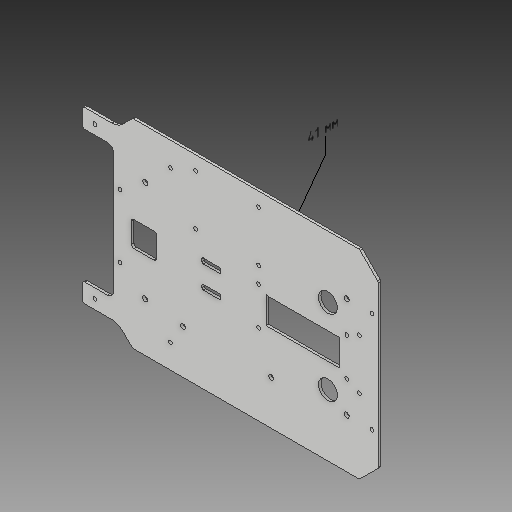
# Autodesk Inventor part: baseUp
Saved by Autodesk Inventor 2019 (Build 230136000, 136)
## iProperties
Created: 2018-05-21
Part Number: baseUp
Material: Типовые
Document SubType Name: Modeling
Designer: olege
Density: 1 g/cm^3
Appearance: По умолчанию
Mass: 63.0766 g
Surface Area: 659.094 cm^2
Volume: 63.0766 cm^3
Author: olege
Autodesk Inventor part; units mm, degrees
ref_plane "YZ Plane" through (0, 0, 0) normal (1, 0, 0) x (0, 1, 0)
ref_plane "XZ Plane" through (0, 0, 0) normal (0, 1, 0) x (-1, 0, 0)
sketch "Эскиз1" plane through (0, 0, 0) normal (0, 0, 1) x (1, 0, 0)
  line L0 (105, -79) -> (-105, -79)
  line L1 (-105, -79) -> (-105, 79)
  line L2 (-105, 79) -> (105, 79)
  line L3 (105, 79) -> (105, -79)
  line L4 (105, -79) -> (-105, 79) construction
  line L5 (-105, -79) -> (105, 79) construction
  point P0 (0, 0)
  dimension "d0" = 210
  dimension "d1" = 158
  constraints: 12 end point, 2 midpoint, 2 parallel, 1 horizontal, 1 perpendicular
  measures "d0" distance of L1.end L2.end
  measures "d1" distance of L0.end L1.end
extrude "Выдавливание1" add sketch "Эскиз1" along normal blind 2
chamfer "Фаска1" distance 15 angle 45 4 edges at (105, -79, 1) (-105, -79, 1) (-105, 79, 1) (105, 79, 1)
fillet "Сопряжение1" radius 2 8 edges at (90, 79, 1) (105, 64, 1) (105, -64, 1) (90, -79, 1) (-90, -79, 1) (-105, -64, 1) (-90, 79, 1) (-105, 64, 1)
sketch "Эскиз2" plane through (0, 0, 2) normal (0, 0, 1) x (1, 0, 0)
  line L0 (-100, 40) -> (100, 40) construction
  line L1 (100, 40) -> (100, -40) construction
  line L2 (100, -40) -> (-100, -40) construction
  line L3 (-100, -40) -> (-100, 40) construction
  line L4 (-100, 40) -> (100, -40) construction
  line L5 (100, 40) -> (-100, -40) construction
  circle A0 centre (100, -40) radius 1.5
  circle A1 centre (100, 40) radius 1.5
  point P0 (0, 0)
  dimension "d8" = 200
  dimension "d9" = 80
  dimension "d10" = 3
  dimension "d13" = 3
  constraints: 12 end point, 2 centre point, 2 coincident, 2 midpoint, 2 parallel, 1 horizontal, 1 perpendicular
  measures "d8" distance of L1.end L2.end
  measures "d9" distance of L0.end L1.end
  measures "d10" diameter of A0
  measures "d13" diameter of A1
extrude "фонарь" cut sketch "Эскиз2" against normal blind 2
sketch "Эскиз3" plane through (0, 0, 2) normal (0, 0, 1) x (1, 0, 0)
  line L0 (-90, 20) -> (90, 20) construction
  line L1 (90, 20) -> (90, -20) construction
  line L2 (90, -20) -> (-90, -20) construction
  line L3 (-90, -20) -> (-90, 20) construction
  line L4 (-90, 20) -> (90, -20) construction
  line L5 (90, 20) -> (-90, -20) construction
  circle A0 centre (90, -20) radius 1.5
  circle A1 centre (90, 20) radius 1.5
  point P0 (0, 0)
  dimension "d16" = 180
  dimension "d17" = 40
  dimension "d18" = 3
  dimension "d19" = 3
  constraints: 12 end point, 2 centre point, 2 coincident, 2 midpoint, 2 parallel, 1 horizontal, 1 perpendicular
  measures "d16" distance of L1.end L2.end
  measures "d17" distance of L0.end L1.end
  measures "d18" diameter of A0
  measures "d19" diameter of A1
extrude "камера" cut sketch "Эскиз3" against normal blind 2
sketch "Эскиз4" plane through (0, 0, 2) normal (0, 0, 1) x (1, 0, 0)
  line L0 (-80, 40) -> (80, 40) construction
  line L1 (80, 40) -> (80, -40) construction
  line L2 (80, -40) -> (-80, -40) construction
  line L3 (-80, -40) -> (-80, 40) construction
  line L4 (-80, 40) -> (80, -40) construction
  line L5 (80, 40) -> (-80, -40) construction
  circle A0 centre (80, -40) radius 2
  circle A1 centre (-80, -40) radius 2
  circle A2 centre (-80, 40) radius 2
  circle A3 centre (80, 40) radius 2
  point P0 (0, 0)
  dimension "d22" = 160
  dimension "d23" = 80
  dimension "d24" = 4
  dimension "d25" = 4
  dimension "d26" = 4
  dimension "d27" = 4
  constraints: 12 end point, 4 centre point, 4 coincident, 2 midpoint, 2 parallel, 1 horizontal, 1 perpendicular
  measures "d22" distance of L1.end L2.end
  measures "d23" distance of L0.end L1.end
  measures "d24" diameter of A0
  measures "d25" diameter of A1
  measures "d26" diameter of A2
  measures "d27" diameter of A3
extrude "крепление" cut sketch "Эскиз4" against normal blind 2
sketch "Эскиз6" plane through (0, 0, 2) normal (0, 0, 1) x (1, 0, 0)
  line L0 (-40, 68) -> (10, 68) construction
  line L1 (10, 68) -> (10, 28) construction
  line L2 (10, 28) -> (-40, 28) construction
  line L3 (-40, 28) -> (-40, 68) construction
  line L4 (-40, 68) -> (10, 28) construction
  line L5 (10, 68) -> (-40, 28) construction
  line L6 (-105, 63.1716) -> (-105, -63.1716) construction
  circle A0 centre (-80, 40) radius 2 construction
  circle A1 centre (10, 28) radius 1.5
  circle A2 centre (-40, 28) radius 1.5
  circle A3 centre (-40, 68) radius 1.5
  circle A4 centre (10, 68) radius 1.5
  point P0 (0, 0)
  point P1 (-15, 48)
  dimension "d46" = 50
  dimension "d47" = 40
  dimension "d48" = 65
  dimension "d49" = 30
  dimension "d50" = 3
  dimension "d51" = 3
  dimension "d52" = 3
  dimension "d53" = 3
  constraints: 12 end point, 4 centre point, 4 coincident, 2 midpoint, 2 parallel, 1 horizontal, 1 perpendicular
  measures "d46" distance of L1.end L2.end
  measures "d47" distance of L0.end L1.end
  measures "d48" distance between parallel lines of L6 L3
  measures "d50" diameter of A1
  measures "d51" diameter of A2
  measures "d52" diameter of A3
  measures "d53" diameter of A4
extrude "Bullet" cut sketch "Эскиз6" against normal blind 10
sketch "Эскиз7" plane through (0, 0, 0) normal (0, 0, -1) x (-1, 0, 0)
  line L0 (105, -63.1716) -> (105, 63.1716) construction
  circle A0 centre (-20, -44) radius 2
  circle A1 centre (50, -44) radius 2
  line L1 (-89.1716, -79) -> (89.1716, -79) projected
  circle A2 centre (80, -40) radius 2 projected
  point P0 (0, 0)
  dimension "d58" = 4
  dimension "d59" = 4
  dimension "d153" = 35
  dimension "d154" = 35
  dimension "d155" = 55
  dimension "d156" = 70
  constraints: 2 centre point
  measures "d58" diameter of A0
  measures "d59" diameter of A1
  measures "d153" distance from line of L1 A1.centre
  measures "d154" distance from line of L1 A0.centre
  measures "d155" distance from line of L0 A1.centre
  measures "d156" distance of A0.centre A1.centre
extrude "АКБ" cut sketch "Эскиз7" against normal blind 10 contours A0 | A1
sketch "Эскиз8" plane through (0, 0, 0) normal (0, 0, -1) x (-1, 0, 0)
  line L0 (-100, -25) -> (100, -25) construction
  line L1 (100, -25) -> (100, 25) construction
  line L2 (100, 25) -> (-100, 25) construction
  line L3 (-100, 25) -> (-100, -25) construction
  line L4 (-100, -25) -> (100, 25) construction
  line L5 (100, -25) -> (-100, 25) construction
  circle A0 centre (100, 25) radius 1.5
  circle A1 centre (100, -25) radius 1.5
  point P0 (0, 0)
  dimension "d65" = 200
  dimension "d66" = 50
  dimension "d67" = 3
  dimension "d68" = 3
  constraints: 12 end point, 2 centre point, 2 coincident, 2 midpoint, 2 parallel, 1 horizontal, 1 perpendicular
  measures "d65" distance of L2.end L1.end
  measures "d66" distance of L1.end L0.end
  measures "d67" diameter of A0
  measures "d68" diameter of A1
extrude "Дисплей" cut sketch "Эскиз8" against normal blind 10
sketch "Эскиз9" plane through (0, 0, 0) normal (0, 0, -1) x (-1, 0, 0)
  line L0 (-24.5, -10.5) -> (-65.5, 10.5) construction
  line L1 (-65.5, -10.5) -> (-24.5, 10.5) construction
  line L2 (-10, -15) -> (-80, -15) construction
  line L3 (-80, -15) -> (-80, 15) construction
  line L4 (-80, 15) -> (-10, 15) construction
  line L5 (-10, 15) -> (-10, -15) construction
  line L6 (-10, -15) -> (-80, 15) construction
  line L7 (-80, -15) -> (-10, 15) construction
  circle A0 centre (-80, 40) radius 2 construction
  circle A1 centre (-80, 15) radius 1.5
  circle A2 centre (-80, -15) radius 1.5
  circle A3 centre (-10, -15) radius 1.5
  circle A4 centre (-10, 15) radius 1.5
  line L8 (-74, 10.5) -> (-16, 10.5)
  line L9 (-16, 10.5) -> (-16, -10.5)
  line L10 (-16, -10.5) -> (-74, -10.5)
  line L11 (-74, -10.5) -> (-74, 10.5)
  line L12 (-74, 10.5) -> (-16, -10.5) construction
  line L13 (-16, 10.5) -> (-74, -10.5) construction
  point P0 (0, 0)
  point P1 (-45, 0)
  point P2 (-45, 0)
  dimension "d71" = 41
  dimension "d72" = 21
  dimension "d73" = 70
  dimension "d74" = 30
  dimension "d75" = 0
  dimension "d76" = 3
  dimension "d77" = 3
  dimension "d78" = 3
  dimension "d79" = 3
  dimension "d82" = 41
  dimension "d157" = 58
  dimension "d158" = 21
  constraints: 28 end point, 7 midpoint, 4 centre point, 4 coincident, 4 parallel, 2 horizontal, 2 perpendicular, 1 horizontal alignment
  measures "d71" distance of L0.end L1.end
  measures "d72" distance of L1.start L0.end
  measures "d73" distance of L3.end L4.end
  measures "d74" distance of L2.end L3.end
  measures "d75" horizontal distance of A0.centre L3.end
  measures "d76" diameter of A1
  measures "d77" diameter of A2
  measures "d78" diameter of A3
  measures "d79" diameter of A4
  measures "d82" distance of L0.start L1.start
  measures "d157" distance of L9.end L10.end
  measures "d158" distance of L8.end L9.end
extrude "Серво" cut sketch "Эскиз9" against normal blind 10
sketch "Эскиз10" plane through (0, 0, 0) normal (0, 0, -1) x (-1, 0, 0)
  line L0 (91, -10) -> (71, -10)
  line L1 (71, -10) -> (71, 10)
  line L2 (71, 10) -> (91, 10)
  line L3 (91, 10) -> (91, -10)
  line L4 (91, -10) -> (71, 10) construction
  line L5 (71, -10) -> (91, 10) construction
  line L6 (105, -63.1716) -> (105, 63.1716) projected
  point P0 (0, 0)
  point P1 (81, 0)
  point P2 (81, 0)
  dimension "d88" = 20
  dimension "d89" = 20
  dimension "d90" = 14
  constraints: 12 end point, 3 midpoint, 2 parallel, 1 horizontal, 1 horizontal alignment, 1 perpendicular
  measures "d88" distance of L1.end L2.end
  measures "d89" distance of L0.end L1.end
  measures "d90" distance between parallel lines of L6 L3
extrude "Для кабелей" cut sketch "Эскиз10" against normal blind 10
fillet "Сопряжение3" radius 2 4 edges at (-71, 10, 1) (-71, -10, 1) (-91, -10, 1) (-91, 10, 1)
sketch "Эскиз11" plane through (0, 0, 0) normal (0, 0, -1) x (-1, 0, 0)
  line L0 (70, -60) -> (120, -60) construction
  circle A0 centre (120, -60) radius 1.5
  line L1 (105, -63.1716) -> (105, 63.1716) projected
  circle A1 centre (80, -40) radius 2 projected
  line L2 (130, -67.5) -> (60, -67.5)
  line L3 (60, -67.5) -> (60, -52.5)
  line L4 (60, -52.5) -> (130, -52.5)
  line L5 (130, -52.5) -> (130, -67.5)
  line L6 (130, -67.5) -> (60, -52.5) construction
  line L7 (60, -67.5) -> (130, -52.5) construction
  circle A2 centre (60, -60) radius 1.5
  point P0 (0, 0)
  point P1 (95, -60)
  dimension "d94" = 50
  dimension "d96" = 3
  dimension "d98" = 20
  dimension "d99" = 70
  dimension "d100" = 15
  dimension "d126" = 3
  dimension "d127" = 60
  dimension "d128" = 25
  constraints: 14 end point, 3 midpoint, 2 centre point, 2 horizontal, 2 parallel, 1 coincident, 1 perpendicular, 1 point on line
  measures "d94" distance of L0.start L0.end
  measures "d96" diameter of A0
  measures "d98" vertical distance of L0.start A1.centre
  measures "d99" distance of L3.end L4.end
  measures "d100" distance of L2.end L3.end
  measures "d126" diameter of A2
  measures "d127" distance of A2.centre L0.end
  measures "d128" distance between parallel lines of L5 L1
extrude "Выдавливание10" add sketch "Эскиз11" against normal blind 2 contours L2 L3 A2 L4 L5 | L3 A2 picked at (60.1113, -59.5125)
extrude "Выдавливание11" cut sketch "Эскиз11" against normal blind 2 contours A2 L3 | L3 A2
fillet "Сопряжение4" radius 2 2 edges at (-130, -52.5, 1) (-130, -67.5, 1)
fillet "Сопряжение5" radius 12 1 edges at (-101.5, -67.5, 1)
fillet "Сопряжение6" radius 5 1 edges at (-105, -52.5, 1)
ref_plane "РабПлоскость1" through (24.5, 0, 0) normal (0, 1, 0) x (1, 0, 0)
mirror "Зеркальное отражение1" about plane through (24.5, 0, 0) normal (0, 1, 0) of "Выдавливание10"
mirror "Зеркальное отражение2" about plane through (24.5, 0, 0) normal (0, 1, 0) of "Выдавливание11"
mirror "Зеркальное отражение3" about plane through (24.5, 0, 0) normal (0, 1, 0) of "Сопряжение4", "Сопряжение5", "Сопряжение6"
sketch "Эскиз13" plane through (0, 0, 0) normal (0, 0, -1) x (-1, 0, 0)
  line L0 (20, 11) -> (35, 11)
  line L1 (35, 11) -> (35, 7)
  line L2 (35, 7) -> (20, 7)
  line L3 (20, 7) -> (20, 11)
  line L4 (20, -7) -> (35, -7)
  line L5 (35, -7) -> (35, -11)
  line L6 (35, -11) -> (20, -11)
  line L7 (20, -11) -> (20, -7)
  line L8 (105, -47.5) -> (105, 47.5) projected
  point P0 (0, 0)
  point P1 (105, -63.1716)
  point P2 (105, 63.1716)
  dimension "d108" = 15
  dimension "d109" = 4
  dimension "d110" = 15
  dimension "d111" = 4
  dimension "d112" = 7
  dimension "d113" = 7
  dimension "d114" = 70
  constraints: 16 end point, 4 parallel, 2 horizontal, 2 perpendicular, 1 point on line
  measures "d108" distance of L1.end L2.end
  measures "d109" distance of L0.end L1.end
  measures "d110" distance of L5.end L6.end
  measures "d111" distance of L4.end L5.end
  measures "d112" distance from line of point (0, 0) L2
  measures "d113" distance from line of point (0, 0) L4
  measures "d114" distance between parallel lines of L8 L5
extrude "Выдавливание12" cut sketch "Эскиз13" against normal blind 2
fillet "Сопряжение7" radius 1 8 edges at (-20, -7, 1) (-20, 11, 1) (-35, -11, 1) (-35, 7, 1) (-20, -11, 1) (-20, 7, 1) (-35, 11, 1) (-35, -7, 1)
sketch "Эскиз14" plane through (0, 0, 0) normal (0, 0, -1) x (-1, 0, 0)
  circle A0 centre (-65, -30) radius 7.5
  circle A1 centre (-65, 30) radius 7.5
  circle A2 centre (-80, 15) radius 1.5 projected
  circle A3 centre (-80, -15) radius 1.5 projected
  point P0 (0, 0)
  dimension "d118" = 15
  dimension "d119" = 15
  dimension "d120" = 15
  dimension "d121" = 15
  dimension "d122" = 15
  dimension "d123" = 15
  constraints: 2 centre point
  measures "d118" diameter of A0
  measures "d119" diameter of A1
  measures "d120" horizontal distance of A2.centre A1.centre
  measures "d121" horizontal distance of A3.centre A0.centre
  measures "d122" horizontal distance of A3.centre A0.centre
  measures "d123" horizontal distance of A2.centre A1.centre
extrude "Выдавливание13" cut sketch "Эскиз14" against normal blind 2 contours A0 | A1
sketch "Эскиз15" plane through (0, 0, 2) normal (0, 0, 1) x (1, 0, 0)
  line L0 (100, -15) -> (30, -15) construction
  line L1 (30, -15) -> (30, 15) construction
  line L2 (30, 15) -> (100, 15) construction
  line L3 (100, 15) -> (100, -15) construction
  line L4 (100, -15) -> (30, 15) construction
  line L5 (30, -15) -> (100, 15) construction
  line L6 (105, -63.1716) -> (105, 63.1716) construction
  circle A0 centre (100, 15) radius 1.5
  circle A1 centre (30, 15) radius 1.5
  circle A2 centre (30, -15) radius 1.5
  circle A3 centre (100, -15) radius 1.5
  line L7 (85.5, -10.5) -> (44.5, -10.5)
  line L8 (44.5, -10.5) -> (44.5, 10.5)
  line L9 (44.5, 10.5) -> (85.5, 10.5)
  line L10 (85.5, -10.5) -> (44.5, 10.5) construction
  line L11 (44.5, -10.5) -> (85.5, 10.5) construction
  line L12 (90.5, -3.5) -> (85.5, -3.5)
  line L13 (85.5, 3.5) -> (90.5, 3.5)
  line L14 (90.5, 3.5) -> (90.5, -3.5)
  line L15 (90.5, -3.5) -> (80.5, 3.5) construction
  line L16 (80.5, -3.5) -> (90.5, 3.5) construction
  line L17 (85.5, 10.5) -> (85.5, 3.5)
  line L18 (85.5, -3.5) -> (85.5, -10.5)
  point P0 (0, 0)
  point P1 (65, 0)
  point P2 (65, 0)
  point P3 (85.5, 0)
  point P4 (65, 0)
  point P5 (85.5, 0)
  point P6 (85.5, 0)
  dimension "d129" = 70
  dimension "d130" = 30
  dimension "d131" = 5
  dimension "d132" = 3
  dimension "d133" = 3
  dimension "d134" = 3
  dimension "d135" = 3
  dimension "d136" = 41
  dimension "d137" = 21
  dimension "d138" = 10
  dimension "d139" = 7
  dimension "d141" = 7
  dimension "d142" = 7
  dimension "d143" = 41
  dimension "d144" = 7
  constraints: 36 end point, 11 midpoint, 6 parallel, 4 centre point, 4 coincident, 3 horizontal, 2 horizontal alignment, 2 perpendicular, 1 vertical alignment
  measures "d129" distance of L1.end L2.end
  measures "d130" distance of L0.end L1.end
  measures "d131" distance between parallel lines of L6 L3
  measures "d132" diameter of A0
  measures "d133" diameter of A1
  measures "d134" diameter of A2
  measures "d135" diameter of A3
  measures "d136" distance of L8.end L9.end
  measures "d137" distance of L7.end L8.end
  measures "d138" distance of L15.end L13.end
  measures "d139" distance of L16.start L15.end
  measures "d141" distance between parallel lines of L12 L13
  measures "d142" distance of L9.end L13.start
  measures "d143" distance of L7.start L7.end
  measures "d144" distance of L13.end L12.start
sketch "Эскиз16" plane through (0, 0, 2) normal (0, 0, 1) x (1, 0, 0)
  circle A0 centre (100, 15) radius 1.5 projected
  circle A1 centre (80, 15) radius 1.5 projected
  line L0 (100, 16.5) -> (80, 16.5)
  line L1 (80, 16.5) -> (80, 13.5)
  line L2 (80, 13.5) -> (100, 13.5)
  line L3 (100, 13.5) -> (100, 16.5)
  circle A2 centre (100, -15) radius 1.5 projected
  circle A3 centre (80, -15) radius 1.5 projected
  line L4 (100, -13.5) -> (80, -13.5)
  line L5 (80, -13.5) -> (80, -16.5)
  line L6 (80, -16.5) -> (100, -16.5)
  line L7 (100, -16.5) -> (100, -13.5)
  circle A4 centre (30, -15) radius 1.5 projected
  circle A5 centre (10, -15) radius 1.5 projected
  line L8 (30, -13.5) -> (10, -13.5)
  line L9 (10, -13.5) -> (10, -16.5)
  line L10 (10, -16.5) -> (30, -16.5)
  line L11 (30, -16.5) -> (30, -13.5)
  circle A6 centre (30, 15) radius 1.5 projected
  circle A7 centre (10, 15) radius 1.5 projected
  line L12 (30, 16.5) -> (10, 16.5)
  line L13 (10, 16.5) -> (10, 13.5)
  line L14 (10, 13.5) -> (30, 13.5)
  line L15 (30, 13.5) -> (30, 16.5)
  point P0 (0, 0)
  constraints: 32 end point, 8 parallel, 8 vertical alignment, 5 point on line, 4 horizontal, 4 perpendicular, 8 other
equation "\"d119\" = d118"
equation "\"d120\" = d121"
equation "\"d123\" = d122"
